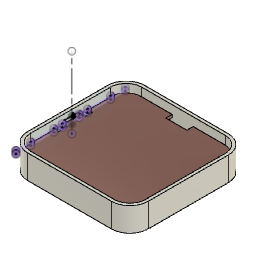
controller_wall_housing (Autodesk Fusion 360 design; units mm, degrees)
Autodesk Fusion 360 part; units mm, degrees
sketch "Sketch1" plane through (0, 0, 0) normal (0, 0, 1) x (1, 0, 0) in component "housing_body"
  line L0 (-19.8989, 27.2279) -> (19.864, 27.2279)
  line L1 (28.664, 18.4279) -> (28.664, -19.5721)
  line L2 (19.864, -28.3721) -> (-19.8989, -28.3721)
  line L3 (-28.6989, -19.5721) -> (-28.6989, 18.4279)
  line L4 (-0.0174, 55) -> (-0.0174, -45)
  line L5 (-50, -0.5721) -> (50, -0.5721)
  arc A0 (-19.8989, 27.2279) -> (-28.6989, 18.4279) centre (-19.8989, 18.4279) ccw
  arc A1 (28.664, 18.4279) -> (19.864, 27.2279) centre (19.864, 18.4279) ccw
  arc A2 (-28.6989, -19.5721) -> (-19.8989, -28.3721) centre (-19.8989, -19.5721) ccw
  arc A3 (19.864, -28.3721) -> (28.664, -19.5721) centre (19.864, -19.5721) ccw
  line L6 (27.264, 18.4279) -> (27.264, -19.5721)
  arc A4 (19.864, -26.9721) -> (27.264, -19.5721) centre (19.864, -19.5721) ccw
  line L7 (19.864, -26.9721) -> (-19.8989, -26.9721)
  arc A5 (-27.2989, -19.5721) -> (-19.8989, -26.9721) centre (-19.8989, -19.5721) ccw
  line L8 (-27.2989, -19.5721) -> (-27.2989, 18.4279)
  arc A6 (-19.8989, 25.8279) -> (-27.2989, 18.4279) centre (-19.8989, 18.4279) ccw
  line L9 (-19.8989, 25.8279) -> (19.864, 25.8279)
  arc A7 (27.264, 18.4279) -> (19.864, 25.8279) centre (19.864, 18.4279) ccw
  circle A8 centre (-11.1774, -12) radius 1.95
  circle A9 centre (11.1426, -12) radius 1.95
  arc A10 (-26.5752, 21.6195) -> (-23.0905, 25.1042) centre (-25.1314, 23.6605) ccw
  arc A11 (23.0556, 25.1042) -> (26.5403, 21.6195) centre (25.0966, 23.6605) ccw
  arc A12 (-23.0905, -26.2484) -> (-26.5752, -22.7637) centre (-25.1314, -24.8047) ccw
  arc A13 (26.5403, -22.7637) -> (23.0556, -26.2484) centre (25.0966, -24.8047) ccw
  point P0 (-28.6989, 27.2279)
  point P1 (-28.6989, -28.3721)
  dimension "d5" = 55.6
  dimension "d6" = 1.4
  dimension "d8" = 8.8
  dimension "d9" = 8.8
  dimension "d17" = 3.9
  dimension "d20" = 5
  dimension "d56" = 22.32
  constraint vertical L1
  constraint horizontal L2
  constraint vertical L3
  constraint horizontal L0
  constraint perpendicular L2 L4
  constraint symmetric L1 L3 L4
  constraint perpendicular L3 L5
  constraint symmetric L0 L2 L5
  constraint coincident P0 L0
  constraint coincident P0 L3
  constraint tangent L0 A0
  constraint tangent L3 A0
  constraint tangent L0 A1
  constraint tangent L1 A1
  constraint equal A0 A1
  constraint coincident P1 L2
  constraint coincident P1 L3
  constraint tangent L2 A2
  constraint tangent L3 A2
  constraint tangent L1 A3
  constraint tangent L2 A3
  constraint equal A2 A3
  constraint equal A8 A9
  constraint symmetric L4 A8 A9
  constraint midpoint A6 A10.centre
  constraint coincident A6 A10.start
  constraint coincident A6 A10.end
  constraint symmetric L4 A10 A11
  constraint symmetric L4 A10.start A11.end
  constraint symmetric L4 A10.end A11.start
  constraint symmetric L5 A10 A12
  constraint symmetric L5 A10.start A12.end
  constraint symmetric L5 A10.end A12.start
  constraint symmetric L5 A11.end A13.start
  constraint symmetric L5 A11.start A13.end
  constraint symmetric L5 A11 A13
  measures "d5" distance of P0 P1
  measures "d8" radius of A0
  measures "d9" radius of A2
  measures "d17" diameter of A8
  measures "d20" diameter of A10
  measures "d56" distance of A8.centre A9.centre
extrude "Extrude1" add sketch "Sketch1" along normal blind 10 contours L0 L3 L4 L5 A0 L8 A6 L9 | L0 L1 L4 L5 A1 L6 L9 A7 | L2 L3 L4 L5 A2 L7 A5 L8 | L1 L2 L4 L5 A3 L6 A4 L7 makes body 1 in component "housing_body"
extrude "Extrude2" add sketch "Sketch1" against normal blind 1.4 contours L4 L5 L6 L9 A7 A11 | L4 L5 L8 A6 L9 A10 | L4 L5 L6 A4 L7 A13 | L4 L5 L7 A5 L8 A12 | A6 A10 | A7 A11 | A5 A12 | A4 A13 bodies 1 in component "housing_body"
extrude "Extrude3" add sketch "Sketch1" along normal blind 5 separate body contours A6 A10 | A7 A11 | A5 A12 | A4 A13 makes body 2 at (26.4383, 21.551, 3.3333) makes body 3 at (-24.9502, -22.3113, 3.3333) makes body 4 at (-23.4077, 21.8498, 3.3333) makes body 5 at (22.7656, -25.7084, 1.6667) in component "housing_body"
combine "Combine1" operation add target body 1 tool bodies 2 3 5 4 in component "housing_body"
sketch "Sketch4" plane through (0, 0, 5) normal (0, 0, 1) x (-1, 0, 0) in component "housing_separator"
  arc A0 (26.5752, -21.6195) -> (23.0905, -25.1042) centre (25.1314, -23.6605) ccw
  arc A1 (23.0905, -25.1042) -> (26.5752, -21.6195) centre (19.8989, -18.4279) ccw
  circle A2 centre (-11.1426, 12) radius 1.95
  circle A3 centre (11.1774, 12) radius 1.95
  line L0 (28.6989, 19.5721) -> (28.6989, -18.4279)
  arc A4 (19.8989, -27.2279) -> (28.6989, -18.4279) centre (19.8989, -18.4279) ccw
  line L1 (19.8989, -27.2279) -> (-19.864, -27.2279)
  arc A5 (-28.664, -18.4279) -> (-19.864, -27.2279) centre (-19.864, -18.4279) ccw
  line L2 (-28.664, -18.4279) -> (-28.664, 19.5721)
  arc A6 (-19.864, 28.3721) -> (-28.664, 19.5721) centre (-19.864, 19.5721) ccw
  line L3 (-19.864, 28.3721) -> (19.8989, 28.3721)
  arc A7 (28.6989, 19.5721) -> (19.8989, 28.3721) centre (19.8989, 19.5721) ccw
  arc A8 (-26.864, -18.4279) -> (-19.864, -25.4279) centre (-19.864, -18.4279) ccw
  arc A9 (19.8989, -25.4279) -> (26.8989, -18.4279) centre (19.8989, -18.4279) ccw
  arc A10 (26.8989, 19.5721) -> (19.8989, 26.5721) centre (19.8989, 19.5721) ccw
  arc A11 (-19.864, 26.5721) -> (-26.864, 19.5721) centre (-19.864, 19.5721) ccw
  line L4 (-4.9826, -25.4279) -> (-4.9826, -22.4279)
  line L5 (-4.9826, -22.4279) -> (5.0174, -22.4279)
  line L6 (5.0174, -22.4279) -> (5.0174, -25.4279)
  line L7 (26.8989, 0.5721) -> (-26.864, 0.5721)
  line L8 (19.8989, -25.4279) -> (5.0174, -25.4279)
  line L9 (-4.9826, -25.4279) -> (-19.864, -25.4279)
  line L10 (0.0174, -27.2279) -> (0.0174, 28.3721)
  line L11 (5.0174, 23.5721) -> (5.0174, 26.5721)
  line L12 (-4.9826, 23.5721) -> (5.0174, 23.5721)
  line L13 (-4.9826, 26.5721) -> (-4.9826, 23.5721)
  line L14 (-19.864, 26.5721) -> (-4.9826, 26.5721)
  line L15 (5.0174, 26.5721) -> (19.8989, 26.5721)
  line L16 (26.8989, -7.4279) -> (24.8989, -7.4279)
  line L17 (24.8989, -7.4279) -> (24.8989, -3.4279)
  line L18 (24.8989, -3.4279) -> (26.8989, -3.4279)
  line L19 (26.8989, -3.4279) -> (26.1989, -3.4279)
  line L20 (26, 4.5721) -> (26.8989, 4.5721)
  line L21 (26.8989, 4.5721) -> (26.8989, -3.4279)
  line L22 (26.8989, -7.4279) -> (26.8989, -18.4279)
  line L23 (24.8989, 4.5721) -> (26.8989, 4.5721)
  line L24 (24.8989, 8.5721) -> (24.8989, 4.5721)
  line L25 (26.8989, 8.5721) -> (24.8989, 8.5721)
  line L26 (26.8989, 19.5721) -> (26.8989, 8.5721)
  line L27 (26.8989, 4.5721) -> (26.8989, -3.4279)
  line L28 (-26.864, -7.4279) -> (-24.864, -7.4279)
  line L29 (-24.864, -7.4279) -> (-24.864, -3.4279)
  line L30 (-24.864, -3.4279) -> (-26.864, -3.4279)
  line L31 (-24.864, 8.5721) -> (-24.864, 4.5721)
  line L32 (-26.864, 8.5721) -> (-24.864, 8.5721)
  line L33 (-24.864, 4.5721) -> (-26.864, 4.5721)
  line L34 (-26.864, -18.4279) -> (-26.864, -7.4279)
  line L35 (-26.864, -3.4279) -> (-26.864, 4.5721)
  line L36 (-26.864, 8.5721) -> (-26.864, 19.5721)
  dimension "d32" = 10
  dimension "d33" = 3
  dimension "d34" = 2
  dimension "d35" = 4
  dimension "d37" = 8
  dimension "d38" = 0.7
  dimension "d39" = 1.8
  constraint vertical L4
  constraint horizontal L5
  constraint vertical L6
  constraint concentric A5 A8
  constraint parallel L1 L8
  constraint concentric A4 A9
  constraint parallel L0 L26
  constraint concentric A7 A10
  constraint parallel L3 L14
  constraint concentric A6 A11
  constraint parallel L2 L34
  constraint tangent A11 L34
  constraint tangent A11 L14
  constraint tangent A10 L14
  constraint tangent A9 L26
  constraint tangent A9 L8
  constraint tangent A8 L8
  constraint tangent A10 L26
  constraint tangent A8 L34
  constraint collinear L8 L9
  constraint equal L8 L9
  constraint midpoint L1 L10.start
  constraint midpoint L3 L10.end
  constraint symmetric L6.end L7 L11.end
  constraint symmetric L4.start L7 L13.start
  constraint symmetric L4.end L7 L12.start
  constraint symmetric L5.end L7 L11.start
  constraint collinear L14 L15
  constraint horizontal L16
  constraint vertical L17
  constraint horizontal L18
  constraint coincident L16.start L26
  constraint horizontal L19
  constraint horizontal L20
  constraint vertical L21
  constraint collinear L22 L26
  constraint coincident L7.start L26
  constraint symmetric L7 L16.start L25.start
  constraint symmetric L7 L16.end L24.start
  constraint symmetric L7 L17.end L23.start
  constraint symmetric L7 L18.end L20.end
  constraint collinear L26 L27
  constraint symmetric L10 L16.start L28.start
  constraint symmetric L10 L16.end L28.end
  constraint symmetric L10 L17.end L29.end
  constraint symmetric L10 L18.end L30.end
  constraint symmetric L10 L23.start L31.end
  constraint symmetric L10 L20.end L33.end
  constraint symmetric L10 L24.start L31.start
  constraint symmetric L10 L25.start L32.start
  constraint collinear L34 L35
  constraint coincident L7.end L34
  constraint collinear L35 L36
  constraint coincident L20.start L23
  measures "d32" distance of L4.end L5.end
  measures "d33" distance of L6.end L5.end
  measures "d34" distance of L16.start L16.end
  measures "d35" distance of L16.start L18.end
  measures "d38" distance of L18.end L19.end
  measures "d39" distance of L1 L8
extrude "Extrude1'" add sketch "Sketch4" along normal blind 1.4 separate body contours A0 A9 | A0 A9 L5 L6 L7 L8 L10 L16 L17 L18 L19 L21 L22 L27 | A8 L4 L5 L7 L9 L10 L28 L29 L30 L34 L35 | A10 L7 L10 L11 L12 L15 L20 L21 L23 L24 L25 L26 L27 | A11 L7 L10 L12 L13 L14 L31 L32 L33 L35 L36 | A2 | A3 makes body 6 in component "housing_separator"
chamfer "Chamfer2" distance 0.7 angle 45 2 edges at (26.864, -0.5721, 6.4) (26.864, -0.5721, 5) on bodies 6 in component "housing_separator"
sketch "Sketch1 (1)" plane through (-27.2989, 0, 0) normal (1, 0, 0) x (0, 1, 0) in component "housing_body"
  line L0 (-19.5721, 0) -> (18.4279, 0)
  line L1 (18.4279, 0) -> (18.4279, 10)
  line L2 (18.4279, 10) -> (-19.5721, 10)
  line L3 (-19.5721, 10) -> (-19.5721, 0)
  line L4 (-3.5, 6) -> (3.5, 6)
  line L5 (3.5, 6) -> (3.5, 7.4)
  line L6 (3.5, 7.4) -> (-3.5, 7.4)
  line L7 (-3.5, 7.4) -> (-3.5, 6)
  line L8 (0, 0) -> (0, 34)
  line L9 (-4.5721, 5.7) -> (3.4279, 5.7)
  line L10 (25.4279, 6.4) -> (18.4279, 6.4)
  line L11 (18.4279, 6.4) -> (7.4279, 6.4)
  line L12 (7.4279, 6.4) -> (3.4279, 6.4)
  line L13 (3.4279, 6.4) -> (-4.5721, 6.4)
  line L14 (-4.5721, 6.4) -> (-8.5721, 6.4)
  line L15 (-8.5721, 6.4) -> (-19.5721, 6.4)
  line L16 (-19.5721, 6.4) -> (-26.5721, 6.4)
  line L17 (-26.5721, 5) -> (-26.5721, 6.4)
  line L18 (-19.5721, 5) -> (-26.5721, 5)
  line L19 (-19.5721, 5) -> (-8.5721, 5)
  line L20 (-8.5721, 5) -> (-4.5721, 5)
  line L21 (-4.5721, 5) -> (3.4279, 5)
  line L22 (7.4279, 5) -> (3.4279, 5)
  line L23 (7.4279, 5) -> (18.4279, 5)
  line L24 (25.4279, 5) -> (18.4279, 5)
  line L25 (25.4279, 5) -> (25.4279, 6.4)
  point P0 (0, 7.4)
  point P1 (0, 4)
  dimension "d44" = 7
  dimension "d45" = 1.4
  dimension "d49" = 0.6
  constraint horizontal L4
  constraint vertical L5
  constraint horizontal L6
  constraint vertical L7
  constraint coincident L8.start origin
  constraint perpendicular L4 L8
  constraint midpoint L6 P0
  constraint coincident L8 P0
  constraint symmetric P0 L9 P1
  measures "d44" distance of L5.end L6.end
  measures "d45" distance of L4 L6
delete_face "DeleteFace1" 2 faces at (26.864, -1.9054, 5.7) (26.6307, 0.7612, 5.9334) on bodies 6 in component "housing_separator"
extrude "Extrude5" add sketch "Sketch1 (1)" along normal blind 0.7 draft -45 separate body contours L4 L5 L8 L12 L13 | L4 L7 L8 L13 | L6 L7 L8 L13 | L5 L6 L8 L12 L13 makes body 7 in component "housing_body"
mirror "Mirror1" about plane through (0, 0, 0) normal (1, 0, 0) of bodies 7 makes body 8 in component "housing_body"
combine "Combine2" operation add target body 1 tool bodies 7 8 in component "housing_body"
chamfer "Chamfer3" distance 1.4 angle 35 1 edges at (27.564, -0.5721, 6.4) measured on face at (-11.6446, 0.7612, 6.4) on bodies 6 in component "housing_separator"
sketch "front_pannel_overlay" plane through (0, 0, -1.4) normal (0, 0, -1) x (1, 0, 0) in component "housing_body"
  circle A0 centre (-11.1774, 12) radius 1.95
  circle A1 centre (11.1426, 12) radius 1.95
  arc A2 (27.264, 19.5721) -> (19.864, 26.9721) centre (19.864, 19.5721) ccw
  line L0 (19.864, 26.9721) -> (-19.8989, 26.9721)
  arc A3 (-19.8989, 26.9721) -> (-27.2989, 19.5721) centre (-19.8989, 19.5721) ccw
  line L1 (-27.2989, 19.5721) -> (-27.2989, -18.4279)
  arc A4 (-27.2989, -18.4279) -> (-19.8989, -25.8279) centre (-19.8989, -18.4279) ccw
  line L2 (-19.8989, -25.8279) -> (19.864, -25.8279)
  arc A5 (19.864, -25.8279) -> (27.264, -18.4279) centre (19.864, -18.4279) ccw
  line L3 (27.264, -18.4279) -> (27.264, 19.5721)
  line L4 (-0.0174, 34.0002) -> (-0.0174, -28.9998)
  line L5 (6.1426, -9.4) -> (16.1426, -9.4)
  line L6 (16.1426, -9.4) -> (16.1426, -13.4)
  line L7 (16.1426, -13.4) -> (6.1426, -13.4)
  line L8 (6.1426, -13.4) -> (6.1426, -9.4)
  line L9 (6.1426, -9.4) -> (16.1426, -13.4) construction
  line L10 (16.1426, -9.4) -> (6.1426, -13.4) construction
  line L11 (-16.1774, -9.4) -> (-16.1774, -13.4)
  line L12 (-16.1774, -13.4) -> (-6.1774, -13.4)
  line L13 (-6.1774, -13.4) -> (-6.1774, -9.4)
  line L14 (-6.1774, -9.4) -> (-16.1774, -9.4)
  line L15 (11.1426, 1.1) -> (14.1737, 6.35)
  line L16 (14.1737, 6.35) -> (8.1115, 6.35)
  line L17 (8.1115, 6.35) -> (11.1426, 1.1)
  line L18 (-0.0174, -55) -> (-0.0174, 45)
  line L19 (-11.1774, 8.1) -> (-14.2085, 2.85)
  line L20 (-14.2085, 2.85) -> (-8.1463, 2.85)
  line L21 (-8.1463, 2.85) -> (-11.1774, 8.1)
  point P0 (11.1426, -11.4)
  point P1 (11.1426, 4.6)
  point P2 (-11.1774, 4.6)
  point P3 (-11.1774, 4.6)
  dimension "d57" = 4
  dimension "d58" = 10
  dimension "d59" = 3.5
  dimension "d60" = 3.5
  dimension "d70" = 7.4
  dimension "d71" = 16
  constraint perpendicular L2 L4
  constraint horizontal L5
  constraint perpendicular L5 L6
  constraint parallel L5 L7
  constraint parallel L6 L8
  constraint coincident L9 P0
  constraint coincident L10 P0
  constraint symmetric L4 L5.start L13.end
  constraint symmetric L4 L5.end L11.start
  constraint symmetric L4 L6.end L11.end
  constraint symmetric L4 L7.end L12.end
  constraint perpendicular L16 L18
  constraint symmetric L4 P1 P3
  constraint coincident P3 P2
  constraint collinear A0.centre P3 L19.start
  constraint collinear A1.centre L15.start P1
  constraint collinear A1.centre P0 P1
  constraint horizontal L20
  measures "d57" distance of L5.end L6.end
  measures "d58" distance of L6.end L7.end
  measures "d59" distance of L15.start P1
  measures "d60" distance of L19.start P3
  measures "d70" distance of A0.centre P3
  measures "d71" distance of P0 P1
extrude "Extrude6" cut sketch "front_pannel_overlay" against normal blind 0.6 contours L5 L6 L7 L8 | L11 L12 L13 L14 | L15 L16 L17 | L19 L20 L21 bodies 1 in component "housing_body"
extrude "Extrude7" add sketch "Sketch1" against normal blind 1.4 contours L0 L3 L4 L5 A0 L8 A6 L9 | L0 L1 L4 L5 A1 L6 L9 A7 | L2 L3 L4 L5 A2 L7 A5 L8 | L1 L2 L4 L5 A3 L6 A4 L7 bodies 1 in component "housing_body"
chamfer "Chamfer2'" distance 0.9333 angle 45 2 edges at (-12.9955, -12.7052, -1.4) (9.3245, -12.7052, -1.4) measured on face at (3.3776, -23.4777, -1.4) measured on face at (3.3776, -23.4777, -1.4) on bodies 1 in component "housing_body"
chamfer "Chamfer1" [rolled back] distance 0.8 rotate angle 30 in component "housing_body"
component "housing_body" placed x (1, 0, 0) y (0, 1, 0) z (0, 0, 1) at (0, 0, 0)
component "housing_separator" placed x (1, 0, 0) y (0, 1, 0) z (0, 0, 1) at (0, 0, 0)
equation "housing_side = 55.8 mm"
equation "tolerance = 0.2 mm"
equation "d5 = housing_side - tolerance"
equation "d6 = wall_thickness"
equation "housing_filet = 8.8 mm"
equation "d8 = housing_filet"
equation "d9 = housing_filet"
equation "housing_hight = 10 mm"
equation "wall_thickness = 1.4 mm"
equation "button_diameter = 3.5 mm"
equation "d17 = button_diameter + 2 * tolerance"
equation "lower_comp_hight = 5 mm"
equation "d25 = housing_hight"
equation "d27 = -wall_thickness"
equation "d29 = lower_comp_hight"
equation "clip_length_half = 4 mm"
equation "d37 = 2 * clip_length_half"
equation "d38 = wall_thickness / 2"
equation "d39 = wall_thickness + 2 * tolerance"
equation "d40 = wall_thickness"
equation "d43 = wall_thickness / 2"
equation "d44 = clip_length_half * 2 - 1 mm"
equation "d45 = wall_thickness"
equation "d49 = 3 * tolerance"
equation "d50 = wall_thickness / 2"
equation "d54 = wall_thickness"
equation "d56 = 2 * housing_side / 5"
equation "d59 = button_diameter"
equation "d60 = button_diameter"
equation "d63 = -wall_thickness"
equation "d68 = wall_thickness / 3 * 2"
